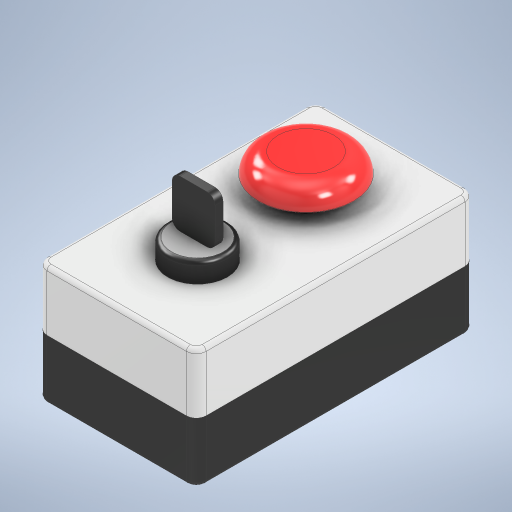
# Autodesk Inventor part: Estop
Saved by Autodesk Inventor 2024 (Build 280153000, 153)
## iProperties
Created: 2023-08-19
Part Number: Estop
Material: Generic
Document SubType Name: Modeling
Designer: 18179
Density: 1 g/cm^3
Appearance: Default
Author: 18179
Autodesk Inventor part; units mm, degrees
ref_plane "YZ Plane" through (0, 0, 0) normal (1, 0, 0) x (0, 1, 0)
ref_plane "XZ Plane" through (0, 0, 0) normal (0, 1, 0) x (-1, 0, 0)
ref_plane "XY Plane" through (0, 0, 0) normal (0, 0, 1) x (1, 0, 0)
sketch "Sketch1" plane through (0, 0, 0) normal (0, 1, 0) x (-1, 0, 0)
  line L0 (3.175, 0) -> (47.625, 0)
  line L1 (50.8, -3.175) -> (50.8, -85.725)
  line L2 (47.625, -88.9) -> (3.175, -88.9)
  line L3 (0, -85.725) -> (0, -3.175)
  arc A0 (50.8, -3.175) -> (47.625, 0) centre (47.625, -3.175) ccw
  arc A1 (47.625, -88.9) -> (50.8, -85.725) centre (47.625, -85.725) ccw
  arc A2 (0, -85.725) -> (3.175, -88.9) centre (3.175, -85.725) ccw
  arc A3 (3.175, 0) -> (0, -3.175) centre (3.175, -3.175) ccw
  point P0 (0, 0)
  point P1 (50.8, -88.9)
  point P2 (50.8, 0)
  point P3 (0, -88.9)
  dimension "d0" = 50.8
  dimension "d1" = 88.9
  dimension "d2" = 3.175
  constraints: 8 end point, 8 point on circle, 8 point on line, 8 tangent, 4 centre point, 3 equal radius, 2 parallel, 1 horizontal, 1 perpendicular
  measures "d0" distance of point (50.8, -88.9) point (0, -88.9)
  measures "d1" distance of point (50.8, 0) point (50.8, -88.9)
  measures "d2" radius of A0
extrude "Extrusion1" add sketch "Sketch1" along normal blind 19.05
sketch "Sketch2" plane through (0, 19.05, 0) normal (0, 1, 0) x (1, 0, 0)
  line L0 (-3.175, 88.9) -> (-47.625, 88.9) projected
  arc A0 (-47.625, 88.9) -> (-50.8, 85.725) centre (-47.625, 85.725) ccw projected
  line L1 (-50.8, 85.725) -> (-50.8, 3.175) projected
  arc A1 (-50.8, 3.175) -> (-47.625, 0) centre (-47.625, 3.175) ccw projected
  line L2 (-47.625, 0) -> (-3.175, 0) projected
  arc A2 (-3.175, 0) -> (0, 3.175) centre (-3.175, 3.175) ccw projected
  line L3 (0, 3.175) -> (0, 85.725) projected
  arc A3 (0, 85.725) -> (-3.175, 88.9) centre (-3.175, 85.725) ccw projected
  line L4 (-50.7746, 3.175) -> (-50.7746, 85.725)
  arc A4 (-47.625, 88.8746) -> (-50.7746, 85.725) centre (-47.625, 85.725) ccw
  line L5 (-47.625, 88.8746) -> (-3.175, 88.8746)
  arc A5 (-0.0254, 85.725) -> (-3.175, 88.8746) centre (-3.175, 85.725) ccw
  line L6 (-0.0254, 85.725) -> (-0.0254, 3.175)
  arc A6 (-3.175, 0.0254) -> (-0.0254, 3.175) centre (-3.175, 3.175) ccw
  line L7 (-3.175, 0.0254) -> (-47.625, 0.0254)
  arc A7 (-50.7746, 3.175) -> (-47.625, 0.0254) centre (-47.625, 3.175) ccw
  point P0 (0, 0)
  dimension "d6" = 0.0254
  constraints: 8 end point, 8 point on circle, 4 centre point, 7 other
  measures "d6" distance between parallel lines of L1 L4
extrude "Extrusion2" add sketch "Sketch2" along normal blind 19.05 contours L4 A4 L5 A5 L6 A6 L7 A7
fillet "Fillet2" radius 1.27 16 edges at (-0.9479, 38.1, -0.9479) (-0.0254, 38.1, -44.45) (-0.9479, 38.1, -87.9521) (-25.4, 38.1, -88.8746) (-49.8521, 38.1, -87.9521) (-50.7746, 38.1, -44.45) (-49.8521, 38.1, -0.9479) (-25.4, 38.1, -0.0254) (-0.9299, 0, -0.9299) (0, 0, -44.45) (-0.9299, 0, -87.9701) (-25.4, 0, -88.9) (-49.8701, 0, -87.9701) (-50.8, 0, -44.45) (-49.8701, 0, -0.9299) (-25.4, 0, 0)
sketch "Sketch3" plane through (0, 38.1, 0) normal (0, 1, 0) x (1, 0, 0)
  line L0 (-3.175, 1.2954) -> (-47.625, 1.2954) projected
  line L1 (-25.4, 1.2954) -> (-25.4, 87.6046)
  line L2 (-47.625, 87.6046) -> (-3.175, 87.6046) projected
  circle A0 centre (-25.4, 60.4005) radius 6.35
  circle A1 centre (-25.4, 25.8016) radius 9.525
  point P0 (0, 0)
  dimension "d10" = 12.7
  dimension "d11" = 19.05
  constraints: 2 centre point, 2 end point, 2 midpoint, 2 point on line
  measures "d10" diameter of A0
  measures "d11" diameter of A1
extrude "Extrusion3" add sketch "Sketch3" along normal blind 6.35
fillet "Fillet3" radius 1.27 1 edges at (-34.925, 44.45, -25.8016)
sketch "Sketch4" plane through (-25.4, 44.45, -60.4005) normal (0, 1, 0) x (1, 0, 0)
  circle A0 centre (0, 0) radius 15.24
  point P0 (25.4, -60.4005)
  dimension "d15" = 30.48
  constraints: 1 centre point
  measures "d15" diameter of A0
extrude "Extrusion4" add sketch "Sketch4" along normal blind 6.35
fillet "Fillet4" radius 6.35 1 edges at (-40.64, 50.8, -60.4005)
fillet "Fillet5" radius 0.254 2 edges at (-40.64, 44.4501, -60.4005) (-40.64, 44.45, -60.4005)
sketch "Sketch5" plane through (-25.4, 44.45, -25.8016) normal (0, 1, 0) x (1, 0, 0)
  circle A0 centre (0, 0) radius 8.255 projected
  line L0 (0, 0) -> (-6.858, 0)
  line L1 (-6.858, 0) -> (-6.858, -1.27)
  line L2 (-6.858, -1.27) -> (0, -1.27)
  line L3 (0, -1.27) -> (0, 0)
  line L4 (-6.858, -1.27) -> (6.858, -1.27)
  line L5 (6.858, -1.27) -> (6.858, 1.27)
  line L6 (6.858, 1.27) -> (-6.858, 1.27)
  line L7 (-6.858, 1.27) -> (-6.858, -1.27)
  point P0 (25.4, -25.8016)
  point P1 (0, -1.27)
  point P2 (-6.858, 0)
  dimension "d20" = 6.858
  dimension "d21" = 1.27
  dimension "d22" = 13.716
  dimension "d23" = 2.54
  constraints: 16 end point, 4 parallel, 2 horizontal, 2 perpendicular
  measures "d20" distance of L2.end L1.end
  measures "d21" distance of L1.end L0.end
  measures "d22" distance of L6.end L5.end
  measures "d23" distance of L5.end L4.end
extrude "Extrusion5" add sketch "Sketch5" along normal blind 15.24 contours L3 L2 L1 L0 | L0 L7 L6 L5 L4 L3
fillet "Fillet6" radius 2.54 2 edges at (-18.542, 59.69, -25.8016) (-32.258, 59.69, -25.8016)
sketch "Sketch6" plane through (-32.258, 44.45, -24.5316) normal (0, 0, 1) x (1, 0, 0)
  arc A0 (2.54, 15.24) -> (0, 12.7) centre (2.54, 12.7) ccw projected
  line L0 (0, 0) -> (0, 12.7) projected
  line L1 (13.716, 0) -> (0, 0) projected
  line L2 (13.716, 0) -> (13.716, 12.7) projected
  arc A1 (13.716, 12.7) -> (11.176, 15.24) centre (11.176, 12.7) ccw projected
  line L3 (2.54, 15.24) -> (11.176, 15.24) projected
  line L4 (0, 0) -> (2.54, 0)
  line L5 (2.54, 0) -> (2.54, 2.54)
  line L6 (2.54, 2.54) -> (0, 2.54)
  line L7 (0, 2.54) -> (0, 0)
  line L8 (13.716, 0) -> (11.176, 0)
  line L9 (11.176, 0) -> (11.176, 2.54)
  line L10 (11.176, 2.54) -> (13.716, 2.54)
  line L11 (13.716, 2.54) -> (13.716, 0)
  circle A2 centre (2.54, 2.54) radius 2.54
  circle A3 centre (11.176, 2.54) radius 2.54
  point P0 (32.258, -44.45)
  point P1 (13.716, 2.54)
  point P2 (0, 2.54)
  dimension "d27" = 2.54
  dimension "d28" = 2.54
  dimension "d29" = 2.54
  dimension "d30" = 2.54
  constraints: 16 end point, 4 parallel, 2 coincident, 2 horizontal, 2 perpendicular, 6 other
  measures "d27" distance of L6.end L5.end
  measures "d28" distance of L5.end L4.end
  measures "d29" distance of L9.end L10.end
  measures "d30" distance of L8.end L9.end
extrude "Extrusion6" cut sketch "Sketch6" against normal blind 15.24 contours A2 L1 L0 | L2 L1 A3
body "Solid1"
